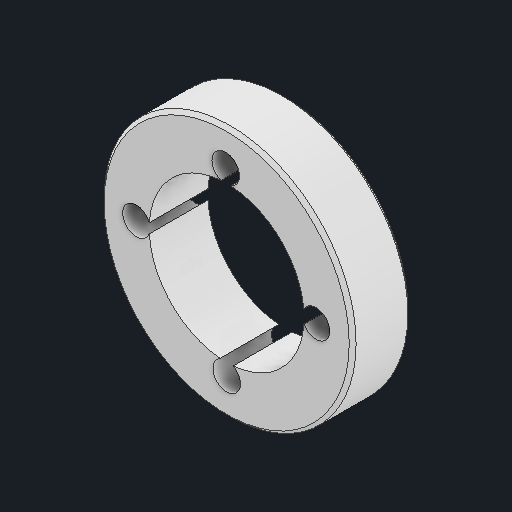
# Autodesk Inventor part: Magnetic
Saved by Autodesk Inventor 2022 (Build 260153070, 153G)
## iProperties
Created: 2021-11-19
Part Number: Magnetic
Material: Типовые
Document SubType Name: Modeling
Designer: kalugin_a
Density: 1 g/cm^3
Appearance: По умолчанию
Author: kalugin_a
Autodesk Inventor part; units mm, degrees
ref_plane "YZ Plane" through (0, 0, 0) normal (1, 0, 0) x (0, 1, 0)
ref_plane "XZ Plane" through (0, 0, 0) normal (0, 1, 0) x (-1, 0, 0)
ref_plane "XY Plane" through (0, 0, 0) normal (0, 0, 1) x (1, 0, 0)
sketch "Эскиз1" plane through (0, 0, 0) normal (0, 0, 1) x (1, 0, 0)
  circle A0 centre (0, 0) radius 22.452
  circle A1 centre (0, 0) radius 36.5
  dimension "d5" = 73
  constraints: 2 centre point, 2 coincident
  measures "d5" diameter of A1
extrude "Выдавливание1" add sketch "Эскиз1" along normal blind 17
chamfer "Фаска1" distance 1 angle 45 2 edges at (-36.5, 0, 0) (-36.5, 0, 17)
sketch "Эскиз2" plane through (0, 0, 17) normal (0, 0, 1) x (1, 0, 0)
  point P0 (-26.1526, -0.0024)
  point P1 (-0.2687, 26.1569)
  point P2 (25.8905, 0.273)
  point P3 (0.0066, -25.8863)
hole "Отверстие1" at (-26.1526, -0.0024, 17) at (-0.2687, 26.1569, 17) at (25.8905, 0.273, 17) at (0.0066, -25.8863, 17) direction (0, 0, -1) diameter 8 end through all
